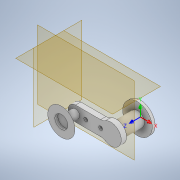
# Autodesk Inventor part: Herramienta1
Saved by Autodesk Inventor 2022 (Build 260153000, 153)
## iProperties
Created: 2022-11-08
Part Number: Herramienta1
Material: Genérico
Document SubType Name: Modeling
Designer: javie
Density: 1 g/cm^3
Appearance: Valor por defecto
Author: javie
Autodesk Inventor part; units mm, degrees
sketch "Boceto1" plane through (0, 0, 0) normal (0, 0, 1) x (1, 0, 0)
  line L0 (85.4549, -45.7257) -> (42.7754, -45.7257)
  line L1 (42.7754, -70.7257) -> (85.4549, -70.7257)
  arc A0 (42.7754, -45.7257) -> (42.7754, -70.7257) centre (42.7754, -58.2257) ccw
  arc A1 (93.4489, -73.0334) -> (93.4489, -43.418) centre (102.7754, -58.2257) ccw
  arc A2 (85.4549, -45.7257) -> (93.4489, -43.418) centre (85.4549, -30.7257) ccw
  arc A3 (93.4489, -73.0334) -> (85.4549, -70.7257) centre (85.4549, -85.7257) ccw
  circle A4 centre (102.7754, -58.2257) radius 8.1
  circle A5 centre (60.2754, -58.2257) radius 3.25
  circle A6 centre (85.4549, -58.2257) radius 3.25
  line L2 (-16.3205, 1) -> (-59, 1)
  line L3 (-59, -24) -> (-16.3205, -24)
  arc A7 (-59, 1) -> (-59, -24) centre (-59, -11.5) ccw
  line L4 (-59, -21.6036) -> (-67.75, -16.5518)
  line L5 (-67.75, -16.5518) -> (-67.75, -6.4482)
  line L6 (-67.75, -6.4482) -> (-59, -1.3964)
  line L7 (-59, -1.3964) -> (-50.25, -6.4482)
  line L8 (-50.25, -6.4482) -> (-50.25, -16.5518)
  line L9 (-50.25, -16.5518) -> (-59, -21.6036)
  arc A8 (-8.3264, -26.3077) -> (-8.3264, 3.3077) centre (1, -11.5) ccw
  arc A9 (-16.3205, 1) -> (-8.3264, 3.3077) centre (-16.3205, 16) ccw
  arc A10 (-8.3264, -26.3077) -> (-16.3205, -24) centre (-16.3205, -39) ccw
  circle A11 centre (1, -11.5) radius 8.1
  circle A12 centre (-41.5, -11.5) radius 3.25
  circle A13 centre (-16.3205, -11.5) radius 3.25
  line L10 (85.6004, 1.2855) -> (42.9209, 1.2855)
  line L11 (42.9209, -23.7145) -> (85.6004, -23.7145)
  arc A14 (42.9209, 1.2855) -> (42.9209, -23.7145) centre (42.9209, -11.2145) ccw
  line L12 (42.9209, -21.3181) -> (34.1709, -16.2663)
  line L13 (34.1709, -16.2663) -> (34.1709, -6.1627)
  line L14 (34.1709, -6.1627) -> (42.9209, -1.1109)
  line L15 (42.9209, -1.1109) -> (51.6709, -6.1627)
  line L16 (51.6709, -6.1627) -> (51.6709, -16.2663)
  line L17 (51.6709, -16.2663) -> (42.9209, -21.3181)
  arc A15 (93.5944, -26.0222) -> (93.5944, 3.5932) centre (102.9209, -11.2145) ccw
  arc A16 (85.6004, 1.2855) -> (93.5944, 3.5932) centre (85.6004, 16.2855) ccw
  arc A17 (93.5944, -26.0222) -> (85.6004, -23.7145) centre (85.6004, -38.7145) ccw
  circle A18 centre (102.9209, -11.2145) radius 8.1
  circle A19 centre (60.4209, -11.2145) radius 3.25
  circle A20 centre (85.6004, -11.2145) radius 3.25
  circle A21 centre (42.7754, -58.2257) radius 7
  line L18 (-15.6185, -45.6026) -> (-58.298, -45.6026)
  line L19 (-58.298, -70.6026) -> (-15.6185, -70.6026)
  arc A22 (-58.298, -45.6026) -> (-58.298, -70.6026) centre (-58.298, -58.1026) ccw
  arc A23 (-7.6244, -72.9103) -> (-7.6244, -43.2949) centre (1.702, -58.1026) ccw
  arc A24 (-15.6185, -45.6026) -> (-7.6244, -43.2949) centre (-15.6185, -30.6026) ccw
  arc A25 (-7.6244, -72.9103) -> (-15.6185, -70.6026) centre (-15.6185, -85.6026) ccw
  circle A26 centre (1.702, -58.1026) radius 8.1
  circle A27 centre (-40.798, -58.1026) radius 3.25
  circle A28 centre (-15.6185, -58.1026) radius 3.25
  circle A29 centre (-58.298, -58.1026) radius 7
  point P0 (90.5279, -45.7257)
  point P1 (90.5279, -70.7257)
  point P2 (-11.2474, 1)
  point P3 (-11.2474, -24)
  point P4 (90.6734, 1.2855)
  point P5 (90.6734, -23.7145)
  point P6 (-10.5454, -45.6026)
  point P7 (-10.5454, -70.6026)
  constraints: 40 end point, 40 point on circle, 30 centre point, 16 tangent, 8 coincident, 8 point on line, 4 equal radius, 4 horizontal, 4 parallel, 26 other
extrude "Extrusión1" add sketch "Boceto1" along normal blind 9 contours A2 A1 A3 L1 A0 L0
sketch "Boceto2" plane through (0, 0, 0) normal (0, 0, -1) x (-1, 0, 0)
  circle A0 centre (-102.7754, -58.2257) radius 8.1 projected
  circle A1 centre (-102.7754, -58.2257) radius 12
  point P0 (0, 0)
  dimension "d13" = 24
  constraints: 2 coincident, 1 centre point
  measures "d13" diameter of A1
extrude "Extrusión2" add sketch "Boceto2" along normal blind 36 and the other way blind 9 contours A0 | A1
sketch "Boceto3" plane through (102.7754, -58.2257, -36) normal (0, 0, -1) x (-1, 0, 0)
  circle A0 centre (0, 0) radius 25
  point P0 (102.7754, 58.2257)
  dimension "d16" = 50
  constraints: 1 centre point
  measures "d16" diameter of A0
extrude "Extrusión3" add sketch "Boceto3" along normal blind 5
ref_plane "Plano de trabajo1" through (42.7754, -58.2257, 0) normal (0, -1, 0) x (1, 0, 0)
sketch "Boceto7" plane through (42.7754, -58.2257, 0) normal (0, -1, 0) x (1, 0, 0)
  line L0 (-7, 0) -> (7, 0) projected
  line L1 (7, 9) -> (7, 0) projected
  line L2 (-7, 0) -> (7, 0)
  line L3 (7, 0) -> (7, 9)
  line L4 (-7, 9) -> (-7, 0)
  line L5 (-7, 9) -> (-7, 22)
  line L6 (7, 22) -> (7, 9)
  line L7 (23, 33) -> (-23, 33)
  line L8 (7, 22) -> (23, 33)
  line L9 (-7, 22) -> (-23, 33)
  line L10 (0, -1.9215) -> (0, 41.7304)
  point P0 (-42.7754, 0)
  point P1 (0, 9)
  point P2 (0, 0)
  point P3 (0, 33)
  dimension "d23" = 14
  dimension "d24" = 13
  dimension "d38" = 46
  dimension "d39" = 11
  constraints: 18 end point, 2 horizontal, 2 parallel, 1 perpendicular, 1 point on line, 1 vertical
  measures "d23" distance of L5.end L6.start
  measures "d24" distance of L5.start L5.end
  measures "d38" distance of L7.start L7.end
  measures "d39" distance from line of L7 L6.start
revolve "Revolución1" add sketch "Boceto7" angle 360 about axis through (42.7754, -58.2257, -1.9215) along (0, 0, 1) contours L4 L5 L9 L7 L10 L0
sketch "Boceto8" plane through (42.7754, -58.2257, 33) normal (0, 0, 1) x (1, 0, 0)
  circle A0 centre (0, 0) radius 11
  point P0 (-42.7754, 58.2257)
  dimension "d29" = 22
  constraints: 1 centre point
  measures "d29" diameter of A0
extrude "Extrusión5" cut sketch "Boceto8" against normal blind 5
